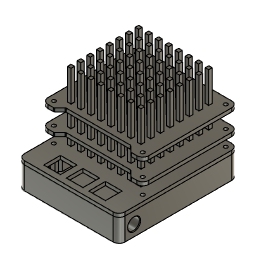
RGB-Audio-Visualiser (Autodesk Fusion 360 design; units mm, degrees)
Autodesk Fusion 360 part; units mm, degrees
sketch "Sketch1" plane through (0, 0, 0) normal (0, 0, 1) x (1, 0, 0) in component "Base"
  line L0 (-42.45, 0) -> (42.45, 0)
  line L1 (42.45, 0) -> (42.45, 100)
  line L2 (42.45, 100) -> (-42.45, 100)
  line L3 (-42.45, 100) -> (-42.45, 0)
  dimension "d18" = 84.9
  dimension "d19" = 100
  constraint horizontal L0
  constraint vertical L1
  constraint horizontal L2
  constraint vertical L3
  constraint midpoint origin L0
  measures "d18" distance of L0.start L0.end
  measures "d19" distance of L0.start L2.end
extrude "Extrude1" add sketch "Sketch1" along normal blind 19 makes body 1 in component "Base"
sketch "Sketch2" plane through (0, 0, 19) normal (0, 0, 1) x (-1, 0, 0) in component "Base"
  line L0 (42.45, -100) -> (42.45, 0)
  line L1 (42.45, 0) -> (-42.45, 0)
  line L2 (-42.45, 0) -> (-42.45, -100)
  line L3 (-42.45, -100) -> (42.45, -100)
  line L4 (33.45, -95) -> (-33.45, -95)
  line L5 (-33.45, -95) -> (-33.45, -5)
  line L6 (-33.45, -5) -> (33.45, -5)
  line L7 (33.45, -5) -> (33.45, -95)
  line L8 (0, -100) -> (0, 0) construction
  line L9 (30.95, -95) -> (-30.95, -95)
  line L10 (-30.95, -95) -> (-30.95, -45)
  line L11 (-33.45, -45) -> (33.45, -45)
  line L12 (30.95, -45) -> (30.95, -95)
  line L13 (-33.45, -21.9) -> (-35.05, -23.5)
  line L14 (-33.45, -21.9) -> (-30.5914, -21.9) construction
  line L15 (-35.05, -23.5) -> (-35.05, -26.5)
  line L16 (-35.05, -26.5) -> (-33.45, -28.1)
  line L17 (-35.05, -25) -> (-42.45, -25) construction
  line L18 (33.45, -21.9) -> (35.05, -23.5)
  line L19 (35.05, -23.5) -> (35.05, -26.5)
  line L20 (35.05, -26.5) -> (33.45, -28.1)
  line L21 (35.05, -25) -> (42.45, -25) construction
  line L22 (33.45, -92.95) -> (30.95, -92.95)
  line L23 (-30.95, -92.95) -> (-33.45, -92.95)
  dimension "d22" = 66.9
  dimension "d23" = 5
  dimension "d24" = 5
  dimension "d25" = 2.5
  dimension "d26" = 50
  dimension "d35" = 135
  dimension "d36" = 3
  dimension "d37" = 1.6
  dimension "d38" = 25
  dimension "d39" = 135
  dimension "d112" = 2.05
  constraint horizontal L4
  constraint vertical L5
  constraint horizontal L6
  constraint vertical L7
  constraint midpoint L3 L8.start
  constraint coincident L8.end origin
  constraint horizontal L9
  constraint vertical L10
  constraint horizontal L11
  constraint vertical L12
  constraint symmetric L8 L10 L12
  constraint collinear L4 L9
  constraint coincident L7 L11.end
  constraint coincident L12.start L11
  constraint coincident L5 L11.start
  constraint coincident L10.end L11
  constraint horizontal L14
  constraint coincident L5 L13.start
  constraint vertical L15
  constraint coincident L5 L16.end
  constraint equal L13 L16
  constraint midpoint L15 L17.start
  constraint coincident L2 L17.end
  constraint perpendicular L2 L17
  constraint coincident L7 L18.start
  constraint parallel L7 L19
  constraint coincident L7 L20.end
  constraint equal L18 L20
  constraint equal L13 L18
  constraint equal L15 L19
  constraint midpoint L19 L21.start
  constraint coincident L0 L21.end
  constraint perpendicular L0 L21
  constraint collinear L17 L21
  constraint coincident L7 L22.start
  constraint coincident L12 L22.end
  constraint perpendicular L12 L22
  constraint coincident L10 L23.start
  constraint coincident L5 L23.end
  constraint perpendicular L5 L23
  constraint collinear L22 L23
  measures "d22" distance of L4.start L4.end
  measures "d23" distance of L3 L4
  measures "d24" distance of L1 L6
  measures "d25" distance of L7 L12
  measures "d26" distance of L4 L11
  measures "d35" angle of L13 L14
  measures "d36" distance of L13.end L15.end
  measures "d37" distance of L5 L15
  measures "d38" distance of L1 L17
  measures "d39" angle of L18 L19
  measures "d112" distance of L4 L22.end
extrude "Extrude2" cut sketch "Sketch2" against normal blind 3.3 contours L4 L9 L10 L11 L12 | L7 L11 L12 L22 | L5 L6 L7 L11 | L5 L10 L11 L23 bodies 1 in component "Base"
extrude "Extrude3" cut sketch "Sketch2" against normal up to surface (17 mm away) contours L4 L9 L10 L11 L12 | L5 L6 L7 L11 | L7 L18 L19 L20 | L5 L13 L15 L16 bodies 1 in component "Base"
sketch "Sketch3" plane through (42.45, 0, 0) normal (1, 0, 0) x (0, 1, 0) in component "Base"
  line L0 (0, 0) -> (100, 0)
  line L1 (100, 0) -> (100, 19)
  line L2 (100, 19) -> (0, 19)
  line L3 (0, 19) -> (0, 0)
  circle A0 centre (12.7, 9.2) radius 5
  line L4 (5, 19) -> (5, 2)
  line L5 (5, 2) -> (21.9, 2)
  line L6 (28.1, 2) -> (45, 2)
  dimension "d31" = 10
  dimension "d32" = 7.7
  dimension "d65" = 7.2
  measures "d31" diameter of A0
  measures "d32" distance of A0.centre L4
  measures "d65" distance of A0.centre L5
extrude "Extrude4" cut sketch "Sketch3" against normal through all contours A0 bodies 1 in component "Base"
sketch "Sketch4" plane through (0, 100, 0) normal (0, 1, 0) x (-1, 0, 0) in component "Base"
  line L0 (-42.45, 0) -> (42.45, 0)
  line L1 (42.45, 0) -> (42.45, 19)
  line L2 (42.45, 19) -> (-42.45, 19)
  line L3 (-42.45, 19) -> (-42.45, 0)
  line L4 (-3.9, 6.1) -> (3.9, 6.1)
  line L5 (3.9, 6.1) -> (3.9, 2)
  line L6 (3.9, 2) -> (-3.9, 2)
  line L7 (-3.9, 2) -> (-3.9, 6.1)
  line L8 (0, 19) -> (0, 0) construction
  line L9 (-30.95, 2) -> (30.95, 2)
  line L10 (-5.9, 0) -> (-5.9, 8.3)
  line L11 (-5.9, 8.3) -> (5.9, 8.3)
  line L12 (5.9, 8.3) -> (5.9, 0)
  dimension "d40" = 7.8
  dimension "d41" = 4.1
  dimension "d115" = 2
  dimension "d116" = 2.2
  constraint horizontal L4
  constraint vertical L5
  constraint horizontal L6
  constraint vertical L7
  constraint midpoint L2 L8.start
  constraint coincident L8.end origin
  constraint symmetric L5 L7 L8
  constraint collinear L6 L9
  constraint coincident L0 L10.start
  constraint perpendicular L0 L10
  constraint perpendicular L10 L11
  constraint coincident L0 L12.end
  constraint perpendicular L0 L12
  constraint symmetric L8 L10 L12
  measures "d40" distance of L4.start L4.end
  measures "d41" distance of L4.start L6.end
  measures "d115" distance of L7 L10
  measures "d116" distance of L4 L11
extrude "Extrude5" cut sketch "Sketch4" against normal blind 2 contours L0 L6 L9 L10 L12 | L4 L5 L7 L9 L10 L11 L12 | L4 L5 L6 L7 L9 bodies 1 in component "Base"
extrude "Extrude6" cut sketch "Sketch4" against normal up to surface (5 mm away) contours L4 L5 L6 L7 L9 bodies 1 in component "Base"
sketch "Sketch5" plane through (0, 0, 0) normal (1, 0, 0) x (0, 1, 0) in component "Base"
  line L0 (48, 2) -> (52, 2)
  line L1 (52, 2) -> (52, 9.4)
  line L2 (52, 9.4) -> (48, 9.4)
  line L3 (48, 9.4) -> (48, 2)
  line L4 (95, 2) -> (45, 2)
  line L5 (52, 7.9) -> (52, 9.4)
  line L6 (52, 6) -> (56.5, 6)
  line L7 (56.5, 6) -> (56.5, 2)
  line L8 (56.5, 2) -> (52, 2)
  line L9 (52, 2) -> (52, 6)
  line L10 (95, 19) -> (95, 2)
  dimension "d49" = 4
  dimension "d50" = 4.5
  dimension "d51" = 43
  dimension "d113" = 4
  dimension "d114" = 7.4
  constraint horizontal L0
  constraint vertical L1
  constraint horizontal L2
  constraint vertical L3
  constraint coincident L0.start L4
  constraint vertical L5
  constraint horizontal L6
  constraint vertical L7
  constraint horizontal L8
  constraint vertical L9
  constraint coincident L4 L7.end
  constraint coincident L1 L6.start
  measures "d49" distance of L6.end L7.end
  measures "d50" distance of L1 L7
  measures "d51" distance of L1 L10
  measures "d113" distance of L1.end L2.end
  measures "d114" distance of L0.start L2.end
extrude "Extrude7" add sketch "Sketch5" along normal mid plane 9 bodies 1 in component "Base"
fillet "Fillet1" radius 5 4 edges at (42.45, 0, 9.5) (42.45, 100, 9.5) (-42.45, 0, 9.5) (-42.45, 100, 9.5) on bodies 1 in component "Base"
fillet "Fillet1" radius 0.5 22 edges at (-33.45, 5, 10.5) (33.45, 5, 10.5) (4.5, 48, 5.7) (4.5, 56.5, 4) (-4.5, 48, 5.7) (-4.5, 56.5, 4) (-4.5, 52, 7.7) (4.5, 52, 7.7) (42.45, 8.0384, 11.0081) (-33.45, 8.0384, 11.0081) (-42.45, 8.0384, 7.3919) (33.45, 8.0384, 7.3919) (-3.9, 95, 4.05) (-3.9, 98, 4.05) (3.9, 95, 4.05) (3.9, 98, 4.05) (-33.45, 92.95, 17.35) (33.45, 92.95, 17.35) (5.9, 100, 4.15) (-5.9, 100, 4.15) (5.9, 98, 4.15) (-5.9, 98, 4.15) on bodies 1 in component "Base"
chamfer "Chamfer1" distance 2.5 angle 45 4 edges at (-30.95, 45, 8.85) (-30.95, 95, 10.5) (30.95, 95, 10.5) (30.95, 45, 8.85) on bodies 1 in component "Base"
sketch "Sketch7" plane through (0, 0, 0) normal (0, 0, -1) x (1, 0, 0) in component "Base"
  arc A0 (-42.45, -95) -> (-37.45, -100) centre (-37.45, -95) ccw
  line L0 (-37.45, -100) -> (-6.4, -100)
  line L1 (-5.4, -98) -> (5.4, -98)
  line L2 (6.4, -100) -> (37.45, -100)
  arc A1 (37.45, -100) -> (42.45, -95) centre (37.45, -95) ccw
  line L3 (42.45, -95) -> (42.45, -5)
  arc A2 (42.45, -5) -> (37.45, 0) centre (37.45, -5) ccw
  line L4 (37.45, 0) -> (-37.45, 0)
  arc A3 (-37.45, 0) -> (-42.45, -5) centre (-37.45, -5) ccw
  line L5 (-42.45, -5) -> (-42.45, -95)
  line L6 (-5.9, -99.5) -> (-5.9, -98.5)
  line L7 (5.9, -98.5) -> (5.9, -99.5)
  arc A4 (-6.4, -100) -> (-5.9, -99.5) centre (-6.4, -99.5) ccw
  arc A5 (-5.4, -98) -> (-5.9, -98.5) centre (-5.4, -98.5) ccw
  arc A6 (5.9, -98.5) -> (5.4, -98) centre (5.4, -98.5) ccw
  arc A7 (5.9, -99.5) -> (6.4, -100) centre (6.4, -99.5) ccw
  point P0 (-37.45, -95)
  point P1 (37.45, -95)
  point P2 (-37.45, -25)
  point P3 (37.45, -25)
  dimension "d66" = 25
  constraint coincident P0 A0.centre
  constraint coincident P1 A1.centre
  constraint horizontal P2 P3
  constraint vertical P0 P2
  constraint vertical P1 P3
  measures "d66" distance of L4 P2
hole "Hole2" at (37.45, 25, 0) at (37.45, 95, 0) at (-37.45, 95, 0) at (-37.45, 25, 0) direction (0, 0, 1) diameter 3.1 end through all counterbore diameter 6 counterbore depth 2 bodies 1 in component "Base"
sketch "Sketch1 (2)" plane through (0, 0, 19) normal (0, 0, 1) x (-1, 0, 0) in component "Cover"
  circle A0 centre (37.45, -95) radius 1.55
  circle A1 centre (-37.45, -25) radius 1.55
  circle A2 centre (-37.45, -95) radius 1.55
  circle A3 centre (37.45, -25) radius 1.55
  arc A4 (37.45, -100) -> (42.45, -95) centre (37.45, -95) ccw
  line L0 (42.45, -95) -> (42.45, -5)
  arc A5 (42.45, -5) -> (37.45, 0) centre (37.45, -5) ccw
  line L1 (37.45, 0) -> (-37.45, 0)
  arc A6 (-37.45, 0) -> (-42.45, -5) centre (-37.45, -5) ccw
  line L2 (-42.45, -5) -> (-42.45, -95)
  arc A7 (-42.45, -95) -> (-37.45, -100) centre (-37.45, -95) ccw
  line L3 (-37.45, -100) -> (37.45, -100)
  line L4 (33.45, -21.9) -> (35.05, -23.5)
  line L5 (35.05, -23.5) -> (35.05, -26.5)
  line L6 (35.05, -26.5) -> (33.45, -28.1)
  line L7 (33.45, -28.1) -> (33.45, -92.45)
  line L8 (28.45, -95) -> (-28.45, -95)
  line L9 (-33.45, -92.45) -> (-33.45, -28.1)
  line L10 (-33.45, -28.1) -> (-35.05, -26.5)
  line L11 (-35.05, -26.5) -> (-35.05, -23.5)
  line L12 (-35.05, -23.5) -> (-33.45, -21.9)
  line L13 (-33.45, -21.9) -> (-33.45, -5.5)
  arc A8 (-32.95, -5) -> (-33.45, -5.5) centre (-32.95, -5.5) ccw
  line L14 (-32.95, -5) -> (32.95, -5)
  arc A9 (33.45, -5.5) -> (32.95, -5) centre (32.95, -5.5) ccw
  line L15 (33.45, -5.5) -> (33.45, -21.9)
  line L16 (32.95, -92.95) -> (30.5, -92.95)
  line L17 (30.5, -92.95) -> (28.45, -95)
  line L18 (-28.45, -95) -> (-30.5, -92.95)
  line L19 (-30.5, -92.95) -> (-32.95, -92.95)
  arc A10 (32.95, -92.95) -> (33.45, -92.45) centre (32.95, -92.45) ccw
  arc A11 (-33.45, -92.45) -> (-32.95, -92.95) centre (-32.95, -92.45) ccw
extrude "Extrude1'" add sketch "Sketch1 (2)" along normal blind 3 separate body contours A4 L0 A5 L1 A6 L2 A7 L3 | L4 L5 L6 L7 L8 L9 L10 L11 L12 L13 A8 L14 A9 L15 L16 L17 L18 L19 A10 A11 makes body 2 in component "Cover"
sketch "Sketch2 (2)" plane through (0, 0, 22) normal (0, 0, 1) x (-1, 0, 0) in component "Cover"
  circle A0 centre (-37.45, -25) radius 1.55
  circle A1 centre (-37.45, -95) radius 1.55
  circle A2 centre (37.45, -25) radius 1.55
  circle A3 centre (37.45, -95) radius 1.55
  line L0 (-37.45, -100) -> (37.45, -100)
  arc A4 (37.45, -100) -> (42.45, -95) centre (37.45, -95) ccw
  line L1 (42.45, -95) -> (42.45, -5)
  arc A5 (42.45, -5) -> (37.45, 0) centre (37.45, -5) ccw
  line L2 (37.45, 0) -> (-37.45, 0)
  arc A6 (-37.45, 0) -> (-42.45, -5) centre (-37.45, -5) ccw
  line L3 (-42.45, -5) -> (-42.45, -95)
  arc A7 (-42.45, -95) -> (-37.45, -100) centre (-37.45, -95) ccw
  line L4 (0, -100) -> (0, 0) construction
  line L5 (7, -5) -> (-7, -5)
  line L6 (-7, -5) -> (-7, -19)
  line L7 (-7, -19) -> (7, -19)
  line L8 (7, -19) -> (7, -5)
  line L9 (31.85, -90.85) -> (-31.85, -90.85) construction
  line L10 (-31.85, -90.85) -> (-31.85, -29.15) construction
  line L11 (-31.85, -29.15) -> (31.85, -29.15) construction
  line L12 (31.85, -29.15) -> (31.85, -90.85) construction
  line L13 (37.45, -95) -> (-37.45, -25) construction
  line L14 (-31.85, -90.85) -> (31.85, -29.15) construction
  line L15 (31, -90) -> (28, -90)
  line L16 (28, -90) -> (28, -87)
  line L17 (28, -87) -> (31, -87)
  line L18 (31, -87) -> (31, -90)
  dimension "d77" = 14
  dimension "d78" = 5
  dimension "d79" = 63.7
  dimension "d80" = 61.7
  dimension "d81" = 3
  dimension "d82" = 0.85
  dimension "d83" = 0.85
  constraint midpoint L0 L4.start
  constraint coincident L4.end origin
  constraint horizontal L5
  constraint vertical L6
  constraint horizontal L7
  constraint vertical L8
  constraint equal L5 L8
  constraint symmetric L4 L6 L8
  constraint horizontal L9
  constraint vertical L10
  constraint horizontal L11
  constraint vertical L12
  constraint coincident A3.centre A4.centre
  constraint coincident A0.centre L13.end
  constraint midpoint L13 L14
  constraint horizontal L15
  constraint vertical L16
  constraint horizontal L17
  constraint vertical L18
  constraint equal L15 L18
  measures "d77" distance of L5.start L5.end
  measures "d78" distance of L2 L5
  measures "d79" distance of L9.start L9.end
  measures "d80" distance of L9.end L10.end
  measures "d81" distance of L15.start L15.end
  measures "d82" distance of L9 L15
  measures "d83" distance of L12 L18
extrude "Extrude2'" cut sketch "Sketch2 (2)" against normal through all contours L5 L6 L7 L8 bodies 2 in component "Cover"
pattern_linear "R-Pattern1" count 3 spacing 19 along (-1, 0, 0) both ways of "Extrude2'" in component "Cover"
extrude "Extrude3'" cut sketch "Sketch2 (2)" against normal through all contours L15 L16 L17 L18 bodies 2 in component "Cover"
pattern_linear "R-Pattern2" count 8 spacing 8.4286 along (1, 0, 0) count 8 spacing 8.1429 along (0, -1, 0) of "Extrude3'" in component "Cover"
ref_plane "WorkPlane1" through (0, 50, 32) normal (0, 0, 1) x (-1, 0, 0) in component "Layer"
sketch "Sketch1 (3)" plane through (0, 50, 32) normal (0, 0, 1) x (1, 0, 0) in component "Layer"
  line L0 (28, -20) -> (28, -17)
  line L1 (28, -17) -> (31, -17)
  line L2 (31, -17) -> (31, -20)
  line L3 (31, -20) -> (28, -20)
  line L4 (19.5714, -20) -> (19.5714, -17)
  line L5 (19.5714, -17) -> (22.5714, -17)
  line L6 (22.5714, -17) -> (22.5714, -20)
  line L7 (22.5714, -20) -> (19.5714, -20)
  line L8 (11.1429, -20) -> (11.1429, -17)
  line L9 (11.1429, -17) -> (14.1429, -17)
  line L10 (14.1429, -17) -> (14.1429, -20)
  line L11 (14.1429, -20) -> (11.1429, -20)
  line L12 (2.7143, -20) -> (2.7143, -17)
  line L13 (2.7143, -17) -> (5.7143, -17)
  line L14 (5.7143, -17) -> (5.7143, -20)
  line L15 (5.7143, -20) -> (2.7143, -20)
  line L16 (-5.7143, -20) -> (-5.7143, -17)
  line L17 (-5.7143, -17) -> (-2.7143, -17)
  line L18 (-2.7143, -17) -> (-2.7143, -20)
  line L19 (-2.7143, -20) -> (-5.7143, -20)
  line L20 (-14.1429, -20) -> (-14.1429, -17)
  line L21 (-14.1429, -17) -> (-11.1429, -17)
  line L22 (-11.1429, -17) -> (-11.1429, -20)
  line L23 (-11.1429, -20) -> (-14.1429, -20)
  line L24 (-22.5714, -20) -> (-22.5714, -17)
  line L25 (-22.5714, -17) -> (-19.5714, -17)
  line L26 (-19.5714, -17) -> (-19.5714, -20)
  line L27 (-19.5714, -20) -> (-22.5714, -20)
  line L28 (-31, -20) -> (-31, -17)
  line L29 (-31, -17) -> (-28, -17)
  line L30 (-28, -17) -> (-28, -20)
  line L31 (-28, -20) -> (-31, -20)
  line L32 (28, -11.8571) -> (28, -8.8571)
  line L33 (28, -8.8571) -> (31, -8.8571)
  line L34 (31, -8.8571) -> (31, -11.8571)
  line L35 (31, -11.8571) -> (28, -11.8571)
  line L36 (19.5714, -11.8571) -> (19.5714, -8.8571)
  line L37 (19.5714, -8.8571) -> (22.5714, -8.8571)
  line L38 (22.5714, -8.8571) -> (22.5714, -11.8571)
  line L39 (22.5714, -11.8571) -> (19.5714, -11.8571)
  line L40 (11.1429, -11.8571) -> (11.1429, -8.8571)
  line L41 (11.1429, -8.8571) -> (14.1429, -8.8571)
  line L42 (14.1429, -8.8571) -> (14.1429, -11.8571)
  line L43 (14.1429, -11.8571) -> (11.1429, -11.8571)
  line L44 (2.7143, -11.8571) -> (2.7143, -8.8571)
  line L45 (2.7143, -8.8571) -> (5.7143, -8.8571)
  line L46 (5.7143, -8.8571) -> (5.7143, -11.8571)
  line L47 (5.7143, -11.8571) -> (2.7143, -11.8571)
  line L48 (-5.7143, -11.8571) -> (-5.7143, -8.8571)
  line L49 (-5.7143, -8.8571) -> (-2.7143, -8.8571)
  line L50 (-2.7143, -8.8571) -> (-2.7143, -11.8571)
  line L51 (-2.7143, -11.8571) -> (-5.7143, -11.8571)
  line L52 (-14.1429, -11.8571) -> (-14.1429, -8.8571)
  line L53 (-14.1429, -8.8571) -> (-11.1429, -8.8571)
  line L54 (-11.1429, -8.8571) -> (-11.1429, -11.8571)
  line L55 (-11.1429, -11.8571) -> (-14.1429, -11.8571)
  line L56 (-22.5714, -11.8571) -> (-22.5714, -8.8571)
  line L57 (-22.5714, -8.8571) -> (-19.5714, -8.8571)
  line L58 (-19.5714, -8.8571) -> (-19.5714, -11.8571)
  line L59 (-19.5714, -11.8571) -> (-22.5714, -11.8571)
  line L60 (-31, -11.8571) -> (-31, -8.8571)
  line L61 (-31, -8.8571) -> (-28, -8.8571)
  line L62 (-28, -8.8571) -> (-28, -11.8571)
  line L63 (-28, -11.8571) -> (-31, -11.8571)
  line L64 (28, -3.7143) -> (28, -0.7143)
  line L65 (28, -0.7143) -> (31, -0.7143)
  line L66 (31, -0.7143) -> (31, -3.7143)
  line L67 (31, -3.7143) -> (28, -3.7143)
  line L68 (19.5714, -3.7143) -> (19.5714, -0.7143)
  line L69 (19.5714, -0.7143) -> (22.5714, -0.7143)
  line L70 (22.5714, -0.7143) -> (22.5714, -3.7143)
  line L71 (22.5714, -3.7143) -> (19.5714, -3.7143)
  line L72 (11.1429, -3.7143) -> (11.1429, -0.7143)
  line L73 (11.1429, -0.7143) -> (14.1429, -0.7143)
  line L74 (14.1429, -0.7143) -> (14.1429, -3.7143)
  line L75 (14.1429, -3.7143) -> (11.1429, -3.7143)
  line L76 (2.7143, -3.7143) -> (2.7143, -0.7143)
  line L77 (2.7143, -0.7143) -> (5.7143, -0.7143)
  line L78 (5.7143, -0.7143) -> (5.7143, -3.7143)
  line L79 (5.7143, -3.7143) -> (2.7143, -3.7143)
  line L80 (-5.7143, -3.7143) -> (-5.7143, -0.7143)
  line L81 (-5.7143, -0.7143) -> (-2.7143, -0.7143)
  line L82 (-2.7143, -0.7143) -> (-2.7143, -3.7143)
  line L83 (-2.7143, -3.7143) -> (-5.7143, -3.7143)
  line L84 (-14.1429, -3.7143) -> (-14.1429, -0.7143)
  line L85 (-14.1429, -0.7143) -> (-11.1429, -0.7143)
  line L86 (-11.1429, -0.7143) -> (-11.1429, -3.7143)
  line L87 (-11.1429, -3.7143) -> (-14.1429, -3.7143)
  line L88 (-22.5714, -3.7143) -> (-22.5714, -0.7143)
  line L89 (-22.5714, -0.7143) -> (-19.5714, -0.7143)
  line L90 (-19.5714, -0.7143) -> (-19.5714, -3.7143)
  line L91 (-19.5714, -3.7143) -> (-22.5714, -3.7143)
  line L92 (-31, -3.7143) -> (-31, -0.7143)
  line L93 (-31, -0.7143) -> (-28, -0.7143)
  line L94 (-28, -0.7143) -> (-28, -3.7143)
  line L95 (-28, -3.7143) -> (-31, -3.7143)
  line L96 (28, 4.4286) -> (28, 7.4286)
  line L97 (28, 7.4286) -> (31, 7.4286)
  line L98 (31, 7.4286) -> (31, 4.4286)
  line L99 (31, 4.4286) -> (28, 4.4286)
  line L100 (19.5714, 4.4286) -> (19.5714, 7.4286)
  line L101 (19.5714, 7.4286) -> (22.5714, 7.4286)
  line L102 (22.5714, 7.4286) -> (22.5714, 4.4286)
  line L103 (22.5714, 4.4286) -> (19.5714, 4.4286)
  line L104 (11.1429, 4.4286) -> (11.1429, 7.4286)
  line L105 (11.1429, 7.4286) -> (14.1429, 7.4286)
  line L106 (14.1429, 7.4286) -> (14.1429, 4.4286)
  line L107 (14.1429, 4.4286) -> (11.1429, 4.4286)
  line L108 (2.7143, 4.4286) -> (2.7143, 7.4286)
  line L109 (2.7143, 7.4286) -> (5.7143, 7.4286)
  line L110 (5.7143, 7.4286) -> (5.7143, 4.4286)
  line L111 (5.7143, 4.4286) -> (2.7143, 4.4286)
  line L112 (-5.7143, 4.4286) -> (-5.7143, 7.4286)
  line L113 (-5.7143, 7.4286) -> (-2.7143, 7.4286)
  line L114 (-2.7143, 7.4286) -> (-2.7143, 4.4286)
  line L115 (-2.7143, 4.4286) -> (-5.7143, 4.4286)
  line L116 (-14.1429, 4.4286) -> (-14.1429, 7.4286)
  line L117 (-14.1429, 7.4286) -> (-11.1429, 7.4286)
  line L118 (-11.1429, 7.4286) -> (-11.1429, 4.4286)
  line L119 (-11.1429, 4.4286) -> (-14.1429, 4.4286)
  line L120 (-22.5714, 4.4286) -> (-22.5714, 7.4286)
  line L121 (-22.5714, 7.4286) -> (-19.5714, 7.4286)
  line L122 (-19.5714, 7.4286) -> (-19.5714, 4.4286)
  line L123 (-19.5714, 4.4286) -> (-22.5714, 4.4286)
  line L124 (-31, 4.4286) -> (-31, 7.4286)
  line L125 (-31, 7.4286) -> (-28, 7.4286)
  line L126 (-28, 7.4286) -> (-28, 4.4286)
  line L127 (-28, 4.4286) -> (-31, 4.4286)
  line L128 (28, 12.5714) -> (28, 15.5714)
  line L129 (28, 15.5714) -> (31, 15.5714)
  line L130 (31, 15.5714) -> (31, 12.5714)
  line L131 (31, 12.5714) -> (28, 12.5714)
  line L132 (19.5714, 12.5714) -> (19.5714, 15.5714)
  line L133 (19.5714, 15.5714) -> (22.5714, 15.5714)
  line L134 (22.5714, 15.5714) -> (22.5714, 12.5714)
  line L135 (22.5714, 12.5714) -> (19.5714, 12.5714)
  line L136 (11.1429, 12.5714) -> (11.1429, 15.5714)
  line L137 (11.1429, 15.5714) -> (14.1429, 15.5714)
  line L138 (14.1429, 15.5714) -> (14.1429, 12.5714)
  line L139 (14.1429, 12.5714) -> (11.1429, 12.5714)
  line L140 (2.7143, 12.5714) -> (2.7143, 15.5714)
  line L141 (2.7143, 15.5714) -> (5.7143, 15.5714)
  line L142 (5.7143, 15.5714) -> (5.7143, 12.5714)
  line L143 (5.7143, 12.5714) -> (2.7143, 12.5714)
  line L144 (-5.7143, 12.5714) -> (-5.7143, 15.5714)
  line L145 (-5.7143, 15.5714) -> (-2.7143, 15.5714)
  line L146 (-2.7143, 15.5714) -> (-2.7143, 12.5714)
  line L147 (-2.7143, 12.5714) -> (-5.7143, 12.5714)
  line L148 (-14.1429, 12.5714) -> (-14.1429, 15.5714)
  line L149 (-14.1429, 15.5714) -> (-11.1429, 15.5714)
  line L150 (-11.1429, 15.5714) -> (-11.1429, 12.5714)
  line L151 (-11.1429, 12.5714) -> (-14.1429, 12.5714)
  line L152 (-22.5714, 12.5714) -> (-22.5714, 15.5714)
  line L153 (-22.5714, 15.5714) -> (-19.5714, 15.5714)
  line L154 (-19.5714, 15.5714) -> (-19.5714, 12.5714)
  line L155 (-19.5714, 12.5714) -> (-22.5714, 12.5714)
  line L156 (-31, 12.5714) -> (-31, 15.5714)
  line L157 (-31, 15.5714) -> (-28, 15.5714)
  line L158 (-28, 15.5714) -> (-28, 12.5714)
  line L159 (-28, 12.5714) -> (-31, 12.5714)
  line L160 (28, 20.7143) -> (28, 23.7143)
  line L161 (28, 23.7143) -> (31, 23.7143)
  line L162 (31, 23.7143) -> (31, 20.7143)
  line L163 (31, 20.7143) -> (28, 20.7143)
  line L164 (19.5714, 20.7143) -> (19.5714, 23.7143)
  line L165 (19.5714, 23.7143) -> (22.5714, 23.7143)
  line L166 (22.5714, 23.7143) -> (22.5714, 20.7143)
  line L167 (22.5714, 20.7143) -> (19.5714, 20.7143)
  line L168 (11.1429, 20.7143) -> (11.1429, 23.7143)
  line L169 (11.1429, 23.7143) -> (14.1429, 23.7143)
  line L170 (14.1429, 23.7143) -> (14.1429, 20.7143)
  line L171 (14.1429, 20.7143) -> (11.1429, 20.7143)
  line L172 (2.7143, 20.7143) -> (2.7143, 23.7143)
  line L173 (2.7143, 23.7143) -> (5.7143, 23.7143)
  line L174 (5.7143, 23.7143) -> (5.7143, 20.7143)
  line L175 (5.7143, 20.7143) -> (2.7143, 20.7143)
  line L176 (-5.7143, 20.7143) -> (-5.7143, 23.7143)
  line L177 (-5.7143, 23.7143) -> (-2.7143, 23.7143)
  line L178 (-2.7143, 23.7143) -> (-2.7143, 20.7143)
  line L179 (-2.7143, 20.7143) -> (-5.7143, 20.7143)
  line L180 (-14.1429, 20.7143) -> (-14.1429, 23.7143)
  line L181 (-14.1429, 23.7143) -> (-11.1429, 23.7143)
  line L182 (-11.1429, 23.7143) -> (-11.1429, 20.7143)
  line L183 (-11.1429, 20.7143) -> (-14.1429, 20.7143)
  line L184 (-22.5714, 20.7143) -> (-22.5714, 23.7143)
  line L185 (-22.5714, 23.7143) -> (-19.5714, 23.7143)
  line L186 (-19.5714, 23.7143) -> (-19.5714, 20.7143)
  line L187 (-19.5714, 20.7143) -> (-22.5714, 20.7143)
  line L188 (-31, 20.7143) -> (-31, 23.7143)
  line L189 (-31, 23.7143) -> (-28, 23.7143)
  line L190 (-28, 23.7143) -> (-28, 20.7143)
  line L191 (-28, 20.7143) -> (-31, 20.7143)
  line L192 (28, 28.8571) -> (28, 31.8571)
  line L193 (28, 31.8571) -> (31, 31.8571)
  line L194 (31, 31.8571) -> (31, 28.8571)
  line L195 (31, 28.8571) -> (28, 28.8571)
  line L196 (19.5714, 28.8571) -> (19.5714, 31.8571)
  line L197 (19.5714, 31.8571) -> (22.5714, 31.8571)
  line L198 (22.5714, 31.8571) -> (22.5714, 28.8571)
  line L199 (22.5714, 28.8571) -> (19.5714, 28.8571)
  line L200 (11.1429, 28.8571) -> (11.1429, 31.8571)
  line L201 (11.1429, 31.8571) -> (14.1429, 31.8571)
  line L202 (14.1429, 31.8571) -> (14.1429, 28.8571)
  line L203 (14.1429, 28.8571) -> (11.1429, 28.8571)
  line L204 (2.7143, 28.8571) -> (2.7143, 31.8571)
  line L205 (2.7143, 31.8571) -> (5.7143, 31.8571)
  line L206 (5.7143, 31.8571) -> (5.7143, 28.8571)
  line L207 (5.7143, 28.8571) -> (2.7143, 28.8571)
  line L208 (-5.7143, 28.8571) -> (-5.7143, 31.8571)
  line L209 (-5.7143, 31.8571) -> (-2.7143, 31.8571)
  line L210 (-2.7143, 31.8571) -> (-2.7143, 28.8571)
  line L211 (-2.7143, 28.8571) -> (-5.7143, 28.8571)
  line L212 (-14.1429, 28.8571) -> (-14.1429, 31.8571)
  line L213 (-14.1429, 31.8571) -> (-11.1429, 31.8571)
  line L214 (-11.1429, 31.8571) -> (-11.1429, 28.8571)
  line L215 (-11.1429, 28.8571) -> (-14.1429, 28.8571)
  line L216 (-22.5714, 28.8571) -> (-22.5714, 31.8571)
  line L217 (-22.5714, 31.8571) -> (-19.5714, 31.8571)
  line L218 (-19.5714, 31.8571) -> (-19.5714, 28.8571)
  line L219 (-19.5714, 28.8571) -> (-22.5714, 28.8571)
  line L220 (-31, 28.8571) -> (-31, 31.8571)
  line L221 (-31, 31.8571) -> (-28, 31.8571)
  line L222 (-28, 31.8571) -> (-28, 28.8571)
  line L223 (-28, 28.8571) -> (-31, 28.8571)
  line L224 (28, 37) -> (28, 40)
  line L225 (28, 40) -> (31, 40)
  line L226 (31, 40) -> (31, 37)
  line L227 (31, 37) -> (28, 37)
  line L228 (19.5714, 37) -> (19.5714, 40)
  line L229 (19.5714, 40) -> (22.5714, 40)
  line L230 (22.5714, 40) -> (22.5714, 37)
  line L231 (22.5714, 37) -> (19.5714, 37)
  line L232 (11.1429, 37) -> (11.1429, 40)
  line L233 (11.1429, 40) -> (14.1429, 40)
  line L234 (14.1429, 40) -> (14.1429, 37)
  line L235 (14.1429, 37) -> (11.1429, 37)
  line L236 (2.7143, 37) -> (2.7143, 40)
  line L237 (2.7143, 40) -> (5.7143, 40)
  line L238 (5.7143, 40) -> (5.7143, 37)
  line L239 (5.7143, 37) -> (2.7143, 37)
  line L240 (-5.7143, 37) -> (-5.7143, 40)
  line L241 (-5.7143, 40) -> (-2.7143, 40)
  line L242 (-2.7143, 40) -> (-2.7143, 37)
  line L243 (-2.7143, 37) -> (-5.7143, 37)
  line L244 (-14.1429, 37) -> (-14.1429, 40)
  line L245 (-14.1429, 40) -> (-11.1429, 40)
  line L246 (-11.1429, 40) -> (-11.1429, 37)
  line L247 (-11.1429, 37) -> (-14.1429, 37)
  line L248 (-22.5714, 37) -> (-22.5714, 40)
  line L249 (-22.5714, 40) -> (-19.5714, 40)
  line L250 (-19.5714, 40) -> (-19.5714, 37)
  line L251 (-19.5714, 37) -> (-22.5714, 37)
  line L252 (-31, 37) -> (-31, 40)
  line L253 (-31, 40) -> (-28, 40)
  line L254 (-28, 40) -> (-28, 37)
  line L255 (-28, 37) -> (-31, 37)
  line L256 (-26, -31) -> (-12, -31)
  line L257 (-12, -31) -> (-12, -45)
  line L258 (-12, -45) -> (-26, -45)
  line L259 (-26, -45) -> (-26, -31)
  line L260 (12, -31) -> (26, -31)
  line L261 (26, -31) -> (26, -45)
  line L262 (26, -45) -> (12, -45)
  line L263 (12, -45) -> (12, -31)
  line L264 (-7, -31) -> (7, -31)
  line L265 (7, -31) -> (7, -45)
  line L266 (7, -45) -> (-7, -45)
  line L267 (-7, -45) -> (-7, -31)
  circle A0 centre (37.45, -25) radius 1.55
  circle A1 centre (37.45, 45) radius 1.55
  circle A2 centre (-37.45, -25) radius 1.55
  circle A3 centre (-37.45, 45) radius 1.55
  line L268 (37.45, 50) -> (-37.45, 50)
  arc A4 (-37.45, 50) -> (-42.45, 45) centre (-37.45, 45) ccw
  line L269 (-42.45, 45) -> (-42.45, -45)
  arc A5 (-42.45, -45) -> (-37.45, -50) centre (-37.45, -45) ccw
  line L270 (-37.45, -50) -> (37.45, -50)
  arc A6 (37.45, -50) -> (42.45, -45) centre (37.45, -45) ccw
  line L271 (42.45, -45) -> (42.45, 45)
  arc A7 (42.45, 45) -> (37.45, 50) centre (37.45, 45) ccw
  line L272 (-42.45, -30) -> (-32.45, -30)
  line L273 (-32.45, -30) -> (-27.45, -25)
  line L274 (-27.45, -25) -> (27.45, -25)
  line L275 (27.45, -25) -> (32.45, -30)
  line L276 (32.45, -30) -> (42.45, -30)
  dimension "d98" = 5
  dimension "d99" = 135
  dimension "d100" = 5
  constraint coincident L269 L272.start
  constraint perpendicular L269 L272
  constraint perpendicular L269 L274
  constraint coincident L271 L276.end
  constraint perpendicular L271 L276
  constraint equal L272 L276
  constraint equal L273 L275
  constraint collinear L272 L276
  constraint horizontal A2.centre L273.end
  measures "d98" distance of A2.centre L272
  measures "d99" angle of L273 L274
  measures "d100" horizontal distance of A2.centre L272.end
extrude "Extrude1''" add sketch "Sketch1 (3)" along normal blind 3 separate body contours L268 A4 L269 L271 A7 L272 L273 L274 L275 L276 makes body 3 in component "Layer"
fillet "Fillet1'" radius 5 2 edges at (-42.45, 20, 33.5) (42.45, 20, 33.5) on bodies 3 in component "Layer"
fillet "Fillet1'" radius 1 4 edges at (32.45, 20, 33.5) (-32.45, 20, 33.5) (-27.45, 25, 33.5) (27.45, 25, 33.5) on bodies 3 in component "Layer"
extrude "Extrude1'''" add 1 faces at (-38.6333, 59.1429, 35) along direction (0, 0, 1) blind 3 from surface at 15 separate body on bodies 3 makes body 4 in component "Top"
sketch "Sketch1 (4)" plane through (0, 0, 19) normal (0, 0, -1) x (1, 0, 0) in component "Light Sticks"
  line L0 (28, -33) -> (28, -30)
  line L1 (28, -30) -> (31, -30)
  line L2 (31, -30) -> (31, -33)
  line L3 (31, -33) -> (28, -33)
  line L4 (19.5714, -33) -> (19.5714, -30)
  line L5 (19.5714, -30) -> (22.5714, -30)
  line L6 (22.5714, -30) -> (22.5714, -33)
  line L7 (22.5714, -33) -> (19.5714, -33)
  line L8 (11.1429, -33) -> (11.1429, -30)
  line L9 (11.1429, -30) -> (14.1429, -30)
  line L10 (14.1429, -30) -> (14.1429, -33)
  line L11 (14.1429, -33) -> (11.1429, -33)
  line L12 (2.7143, -33) -> (2.7143, -30)
  line L13 (2.7143, -30) -> (5.7143, -30)
  line L14 (5.7143, -30) -> (5.7143, -33)
  line L15 (5.7143, -33) -> (2.7143, -33)
  line L16 (-5.7143, -33) -> (-5.7143, -30)
  line L17 (-5.7143, -30) -> (-2.7143, -30)
  line L18 (-2.7143, -30) -> (-2.7143, -33)
  line L19 (-2.7143, -33) -> (-5.7143, -33)
  line L20 (-14.1429, -33) -> (-14.1429, -30)
  line L21 (-14.1429, -30) -> (-11.1429, -30)
  line L22 (-11.1429, -30) -> (-11.1429, -33)
  line L23 (-11.1429, -33) -> (-14.1429, -33)
  line L24 (-22.5714, -33) -> (-22.5714, -30)
  line L25 (-22.5714, -30) -> (-19.5714, -30)
  line L26 (-19.5714, -30) -> (-19.5714, -33)
  line L27 (-19.5714, -33) -> (-22.5714, -33)
  line L28 (-31, -33) -> (-31, -30)
  line L29 (-31, -30) -> (-28, -30)
  line L30 (-28, -30) -> (-28, -33)
  line L31 (-28, -33) -> (-31, -33)
  line L32 (28, -41.1429) -> (28, -38.1429)
  line L33 (28, -38.1429) -> (31, -38.1429)
  line L34 (31, -38.1429) -> (31, -41.1429)
  line L35 (31, -41.1429) -> (28, -41.1429)
  line L36 (19.5714, -41.1429) -> (19.5714, -38.1429)
  line L37 (19.5714, -38.1429) -> (22.5714, -38.1429)
  line L38 (22.5714, -38.1429) -> (22.5714, -41.1429)
  line L39 (22.5714, -41.1429) -> (19.5714, -41.1429)
  line L40 (11.1429, -41.1429) -> (11.1429, -38.1429)
  line L41 (11.1429, -38.1429) -> (14.1429, -38.1429)
  line L42 (14.1429, -38.1429) -> (14.1429, -41.1429)
  line L43 (14.1429, -41.1429) -> (11.1429, -41.1429)
  line L44 (2.7143, -41.1429) -> (2.7143, -38.1429)
  line L45 (2.7143, -38.1429) -> (5.7143, -38.1429)
  line L46 (5.7143, -38.1429) -> (5.7143, -41.1429)
  line L47 (5.7143, -41.1429) -> (2.7143, -41.1429)
  line L48 (-5.7143, -41.1429) -> (-5.7143, -38.1429)
  line L49 (-5.7143, -38.1429) -> (-2.7143, -38.1429)
  line L50 (-2.7143, -38.1429) -> (-2.7143, -41.1429)
  line L51 (-2.7143, -41.1429) -> (-5.7143, -41.1429)
  line L52 (-14.1429, -41.1429) -> (-14.1429, -38.1429)
  line L53 (-14.1429, -38.1429) -> (-11.1429, -38.1429)
  line L54 (-11.1429, -38.1429) -> (-11.1429, -41.1429)
  line L55 (-11.1429, -41.1429) -> (-14.1429, -41.1429)
  line L56 (-22.5714, -41.1429) -> (-22.5714, -38.1429)
  line L57 (-22.5714, -38.1429) -> (-19.5714, -38.1429)
  line L58 (-19.5714, -38.1429) -> (-19.5714, -41.1429)
  line L59 (-19.5714, -41.1429) -> (-22.5714, -41.1429)
  line L60 (-31, -41.1429) -> (-31, -38.1429)
  line L61 (-31, -38.1429) -> (-28, -38.1429)
  line L62 (-28, -38.1429) -> (-28, -41.1429)
  line L63 (-28, -41.1429) -> (-31, -41.1429)
  line L64 (28, -49.2857) -> (28, -46.2857)
  line L65 (28, -46.2857) -> (31, -46.2857)
  line L66 (31, -46.2857) -> (31, -49.2857)
  line L67 (31, -49.2857) -> (28, -49.2857)
  line L68 (19.5714, -49.2857) -> (19.5714, -46.2857)
  line L69 (19.5714, -46.2857) -> (22.5714, -46.2857)
  line L70 (22.5714, -46.2857) -> (22.5714, -49.2857)
  line L71 (22.5714, -49.2857) -> (19.5714, -49.2857)
  line L72 (11.1429, -49.2857) -> (11.1429, -46.2857)
  line L73 (11.1429, -46.2857) -> (14.1429, -46.2857)
  line L74 (14.1429, -46.2857) -> (14.1429, -49.2857)
  line L75 (14.1429, -49.2857) -> (11.1429, -49.2857)
  line L76 (2.7143, -49.2857) -> (2.7143, -46.2857)
  line L77 (2.7143, -46.2857) -> (5.7143, -46.2857)
  line L78 (5.7143, -46.2857) -> (5.7143, -49.2857)
  line L79 (5.7143, -49.2857) -> (2.7143, -49.2857)
  line L80 (-5.7143, -49.2857) -> (-5.7143, -46.2857)
  line L81 (-5.7143, -46.2857) -> (-2.7143, -46.2857)
  line L82 (-2.7143, -46.2857) -> (-2.7143, -49.2857)
  line L83 (-2.7143, -49.2857) -> (-5.7143, -49.2857)
  line L84 (-14.1429, -49.2857) -> (-14.1429, -46.2857)
  line L85 (-14.1429, -46.2857) -> (-11.1429, -46.2857)
  line L86 (-11.1429, -46.2857) -> (-11.1429, -49.2857)
  line L87 (-11.1429, -49.2857) -> (-14.1429, -49.2857)
  line L88 (-22.5714, -49.2857) -> (-22.5714, -46.2857)
  line L89 (-22.5714, -46.2857) -> (-19.5714, -46.2857)
  line L90 (-19.5714, -46.2857) -> (-19.5714, -49.2857)
  line L91 (-19.5714, -49.2857) -> (-22.5714, -49.2857)
  line L92 (-31, -49.2857) -> (-31, -46.2857)
  line L93 (-31, -46.2857) -> (-28, -46.2857)
  line L94 (-28, -46.2857) -> (-28, -49.2857)
  line L95 (-28, -49.2857) -> (-31, -49.2857)
  line L96 (28, -57.4286) -> (28, -54.4286)
  line L97 (28, -54.4286) -> (31, -54.4286)
  line L98 (31, -54.4286) -> (31, -57.4286)
  line L99 (31, -57.4286) -> (28, -57.4286)
  line L100 (19.5714, -57.4286) -> (19.5714, -54.4286)
  line L101 (19.5714, -54.4286) -> (22.5714, -54.4286)
  line L102 (22.5714, -54.4286) -> (22.5714, -57.4286)
  line L103 (22.5714, -57.4286) -> (19.5714, -57.4286)
  line L104 (11.1429, -57.4286) -> (11.1429, -54.4286)
  line L105 (11.1429, -54.4286) -> (14.1429, -54.4286)
  line L106 (14.1429, -54.4286) -> (14.1429, -57.4286)
  line L107 (14.1429, -57.4286) -> (11.1429, -57.4286)
  line L108 (2.7143, -57.4286) -> (2.7143, -54.4286)
  line L109 (2.7143, -54.4286) -> (5.7143, -54.4286)
  line L110 (5.7143, -54.4286) -> (5.7143, -57.4286)
  line L111 (5.7143, -57.4286) -> (2.7143, -57.4286)
  line L112 (-5.7143, -57.4286) -> (-5.7143, -54.4286)
  line L113 (-5.7143, -54.4286) -> (-2.7143, -54.4286)
  line L114 (-2.7143, -54.4286) -> (-2.7143, -57.4286)
  line L115 (-2.7143, -57.4286) -> (-5.7143, -57.4286)
  line L116 (-14.1429, -57.4286) -> (-14.1429, -54.4286)
  line L117 (-14.1429, -54.4286) -> (-11.1429, -54.4286)
  line L118 (-11.1429, -54.4286) -> (-11.1429, -57.4286)
  line L119 (-11.1429, -57.4286) -> (-14.1429, -57.4286)
  line L120 (-22.5714, -57.4286) -> (-22.5714, -54.4286)
  line L121 (-22.5714, -54.4286) -> (-19.5714, -54.4286)
  line L122 (-19.5714, -54.4286) -> (-19.5714, -57.4286)
  line L123 (-19.5714, -57.4286) -> (-22.5714, -57.4286)
  line L124 (-31, -57.4286) -> (-31, -54.4286)
  line L125 (-31, -54.4286) -> (-28, -54.4286)
  line L126 (-28, -54.4286) -> (-28, -57.4286)
  line L127 (-28, -57.4286) -> (-31, -57.4286)
  line L128 (28, -65.5714) -> (28, -62.5714)
  line L129 (28, -62.5714) -> (31, -62.5714)
  line L130 (31, -62.5714) -> (31, -65.5714)
  line L131 (31, -65.5714) -> (28, -65.5714)
  line L132 (19.5714, -65.5714) -> (19.5714, -62.5714)
  line L133 (19.5714, -62.5714) -> (22.5714, -62.5714)
  line L134 (22.5714, -62.5714) -> (22.5714, -65.5714)
  line L135 (22.5714, -65.5714) -> (19.5714, -65.5714)
  line L136 (11.1429, -65.5714) -> (11.1429, -62.5714)
  line L137 (11.1429, -62.5714) -> (14.1429, -62.5714)
  line L138 (14.1429, -62.5714) -> (14.1429, -65.5714)
  line L139 (14.1429, -65.5714) -> (11.1429, -65.5714)
  line L140 (2.7143, -65.5714) -> (2.7143, -62.5714)
  line L141 (2.7143, -62.5714) -> (5.7143, -62.5714)
  line L142 (5.7143, -62.5714) -> (5.7143, -65.5714)
  line L143 (5.7143, -65.5714) -> (2.7143, -65.5714)
  line L144 (-5.7143, -65.5714) -> (-5.7143, -62.5714)
  line L145 (-5.7143, -62.5714) -> (-2.7143, -62.5714)
  line L146 (-2.7143, -62.5714) -> (-2.7143, -65.5714)
  line L147 (-2.7143, -65.5714) -> (-5.7143, -65.5714)
  line L148 (-14.1429, -65.5714) -> (-14.1429, -62.5714)
  line L149 (-14.1429, -62.5714) -> (-11.1429, -62.5714)
  line L150 (-11.1429, -62.5714) -> (-11.1429, -65.5714)
  line L151 (-11.1429, -65.5714) -> (-14.1429, -65.5714)
  line L152 (-22.5714, -65.5714) -> (-22.5714, -62.5714)
  line L153 (-22.5714, -62.5714) -> (-19.5714, -62.5714)
  line L154 (-19.5714, -62.5714) -> (-19.5714, -65.5714)
  line L155 (-19.5714, -65.5714) -> (-22.5714, -65.5714)
  line L156 (-31, -65.5714) -> (-31, -62.5714)
  line L157 (-31, -62.5714) -> (-28, -62.5714)
  line L158 (-28, -62.5714) -> (-28, -65.5714)
  line L159 (-28, -65.5714) -> (-31, -65.5714)
  line L160 (28, -73.7143) -> (28, -70.7143)
  line L161 (28, -70.7143) -> (31, -70.7143)
  line L162 (31, -70.7143) -> (31, -73.7143)
  line L163 (31, -73.7143) -> (28, -73.7143)
  line L164 (19.5714, -73.7143) -> (19.5714, -70.7143)
  line L165 (19.5714, -70.7143) -> (22.5714, -70.7143)
  line L166 (22.5714, -70.7143) -> (22.5714, -73.7143)
  line L167 (22.5714, -73.7143) -> (19.5714, -73.7143)
  line L168 (11.1429, -73.7143) -> (11.1429, -70.7143)
  line L169 (11.1429, -70.7143) -> (14.1429, -70.7143)
  line L170 (14.1429, -70.7143) -> (14.1429, -73.7143)
  line L171 (14.1429, -73.7143) -> (11.1429, -73.7143)
  line L172 (2.7143, -73.7143) -> (2.7143, -70.7143)
  line L173 (2.7143, -70.7143) -> (5.7143, -70.7143)
  line L174 (5.7143, -70.7143) -> (5.7143, -73.7143)
  line L175 (5.7143, -73.7143) -> (2.7143, -73.7143)
  line L176 (-5.7143, -73.7143) -> (-5.7143, -70.7143)
  line L177 (-5.7143, -70.7143) -> (-2.7143, -70.7143)
  line L178 (-2.7143, -70.7143) -> (-2.7143, -73.7143)
  line L179 (-2.7143, -73.7143) -> (-5.7143, -73.7143)
  line L180 (-14.1429, -73.7143) -> (-14.1429, -70.7143)
  line L181 (-14.1429, -70.7143) -> (-11.1429, -70.7143)
  line L182 (-11.1429, -70.7143) -> (-11.1429, -73.7143)
  line L183 (-11.1429, -73.7143) -> (-14.1429, -73.7143)
  line L184 (-22.5714, -73.7143) -> (-22.5714, -70.7143)
  line L185 (-22.5714, -70.7143) -> (-19.5714, -70.7143)
  line L186 (-19.5714, -70.7143) -> (-19.5714, -73.7143)
  line L187 (-19.5714, -73.7143) -> (-22.5714, -73.7143)
  line L188 (-31, -73.7143) -> (-31, -70.7143)
  line L189 (-31, -70.7143) -> (-28, -70.7143)
  line L190 (-28, -70.7143) -> (-28, -73.7143)
  line L191 (-28, -73.7143) -> (-31, -73.7143)
  line L192 (28, -81.8571) -> (28, -78.8571)
  line L193 (28, -78.8571) -> (31, -78.8571)
  line L194 (31, -78.8571) -> (31, -81.8571)
  line L195 (31, -81.8571) -> (28, -81.8571)
  line L196 (19.5714, -81.8571) -> (19.5714, -78.8571)
  line L197 (19.5714, -78.8571) -> (22.5714, -78.8571)
  line L198 (22.5714, -78.8571) -> (22.5714, -81.8571)
  line L199 (22.5714, -81.8571) -> (19.5714, -81.8571)
  line L200 (11.1429, -81.8571) -> (11.1429, -78.8571)
  line L201 (11.1429, -78.8571) -> (14.1429, -78.8571)
  line L202 (14.1429, -78.8571) -> (14.1429, -81.8571)
  line L203 (14.1429, -81.8571) -> (11.1429, -81.8571)
  line L204 (2.7143, -81.8571) -> (2.7143, -78.8571)
  line L205 (2.7143, -78.8571) -> (5.7143, -78.8571)
  line L206 (5.7143, -78.8571) -> (5.7143, -81.8571)
  line L207 (5.7143, -81.8571) -> (2.7143, -81.8571)
  line L208 (-5.7143, -81.8571) -> (-5.7143, -78.8571)
  line L209 (-5.7143, -78.8571) -> (-2.7143, -78.8571)
  line L210 (-2.7143, -78.8571) -> (-2.7143, -81.8571)
  line L211 (-2.7143, -81.8571) -> (-5.7143, -81.8571)
  line L212 (-14.1429, -81.8571) -> (-14.1429, -78.8571)
  line L213 (-14.1429, -78.8571) -> (-11.1429, -78.8571)
  line L214 (-11.1429, -78.8571) -> (-11.1429, -81.8571)
  line L215 (-11.1429, -81.8571) -> (-14.1429, -81.8571)
  line L216 (-22.5714, -81.8571) -> (-22.5714, -78.8571)
  line L217 (-22.5714, -78.8571) -> (-19.5714, -78.8571)
  line L218 (-19.5714, -78.8571) -> (-19.5714, -81.8571)
  line L219 (-19.5714, -81.8571) -> (-22.5714, -81.8571)
  line L220 (-31, -81.8571) -> (-31, -78.8571)
  line L221 (-31, -78.8571) -> (-28, -78.8571)
  line L222 (-28, -78.8571) -> (-28, -81.8571)
  line L223 (-28, -81.8571) -> (-31, -81.8571)
  line L224 (28, -90) -> (28, -87)
  line L225 (28, -87) -> (31, -87)
  line L226 (31, -87) -> (31, -90)
  line L227 (31, -90) -> (28, -90)
  line L228 (19.5714, -90) -> (19.5714, -87)
  line L229 (19.5714, -87) -> (22.5714, -87)
  line L230 (22.5714, -87) -> (22.5714, -90)
  line L231 (22.5714, -90) -> (19.5714, -90)
  line L232 (11.1429, -90) -> (11.1429, -87)
  line L233 (11.1429, -87) -> (14.1429, -87)
  line L234 (14.1429, -87) -> (14.1429, -90)
  line L235 (14.1429, -90) -> (11.1429, -90)
  line L236 (2.7143, -90) -> (2.7143, -87)
  line L237 (2.7143, -87) -> (5.7143, -87)
  line L238 (5.7143, -87) -> (5.7143, -90)
  line L239 (5.7143, -90) -> (2.7143, -90)
  line L240 (-5.7143, -90) -> (-5.7143, -87)
  line L241 (-5.7143, -87) -> (-2.7143, -87)
  line L242 (-2.7143, -87) -> (-2.7143, -90)
  line L243 (-2.7143, -90) -> (-5.7143, -90)
  line L244 (-14.1429, -90) -> (-14.1429, -87)
  line L245 (-14.1429, -87) -> (-11.1429, -87)
  line L246 (-11.1429, -87) -> (-11.1429, -90)
  line L247 (-11.1429, -90) -> (-14.1429, -90)
  line L248 (-22.5714, -90) -> (-22.5714, -87)
  line L249 (-22.5714, -87) -> (-19.5714, -87)
  line L250 (-19.5714, -87) -> (-19.5714, -90)
  line L251 (-19.5714, -90) -> (-22.5714, -90)
  line L252 (-31, -90) -> (-31, -87)
  line L253 (-31, -87) -> (-28, -87)
  line L254 (-28, -87) -> (-28, -90)
  line L255 (-28, -90) -> (-31, -90)
  line L256 (-12, -19) -> (-26, -19)
  line L257 (-26, -19) -> (-26, -5)
  line L258 (-26, -5) -> (-12, -5)
  line L259 (-12, -5) -> (-12, -19)
  line L260 (26, -19) -> (12, -19)
  line L261 (12, -19) -> (12, -5)
  line L262 (12, -5) -> (26, -5)
  line L263 (26, -5) -> (26, -19)
  line L264 (7, -19) -> (-7, -19)
  line L265 (-7, -19) -> (-7, -5)
  line L266 (-7, -5) -> (7, -5)
  line L267 (7, -5) -> (7, -19)
  circle A0 centre (37.45, -25) radius 1.55
  circle A1 centre (37.45, -95) radius 1.55
  circle A2 centre (-37.45, -25) radius 1.55
  circle A3 centre (-37.45, -95) radius 1.55
  line L268 (-37.45, -100) -> (37.45, -100)
  arc A4 (37.45, -100) -> (42.45, -95) centre (37.45, -95) ccw
  line L269 (42.45, -95) -> (42.45, -5)
  arc A5 (42.45, -5) -> (37.45, 0) centre (37.45, -5) ccw
  line L270 (37.45, 0) -> (-37.45, 0)
  arc A6 (-37.45, 0) -> (-42.45, -5) centre (-37.45, -5) ccw
  line L271 (-42.45, -5) -> (-42.45, -95)
  arc A7 (-42.45, -95) -> (-37.45, -100) centre (-37.45, -95) ccw
extrude "Extrude1''''" add sketch "Sketch1 (4)" against normal blind 60 separate body contours L0 L1 L2 L3 | L4 L5 L6 L7 | L8 L9 L10 L11 | L12 L13 L14 L15 | L16 L17 L18 L19 | L20 L21 L22 L23 | L24 L25 L26 L27 | L28 L29 L30 L31 | L32 L33 L34 L35 | L36 L37 L38 L39 | L40 L41 L42 L43 | L44 L45 L46 L47 | L48 L49 L50 L51 | L52 L53 L54 L55 | L56 L57 L58 L59 | L60 L61 L62 L63 | L64 L65 L66 L67 | L68 L69 L70 L71 | L72 L73 L74 L75 | L76 L77 L78 L79 | L80 L81 L82 L83 | L84 L85 L86 L87 | L88 L89 L90 L91 | L92 L93 L94 L95 | L96 L97 L98 L99 | L100 L101 L102 L103 | L104 L105 L106 L107 | L108 L109 L110 L111 | L112 L113 L114 L115 | L116 L117 L118 L119 | L120 L121 L122 L123 | L124 L125 L126 L127 | L128 L129 L130 L131 | L132 L133 L134 L135 | L136 L137 L138 L139 | L140 L141 L142 L143 | L144 L145 L146 L147 | L148 L149 L150 L151 | L152 L153 L154 L155 | L156 L157 L158 L159 | L160 L161 L162 L163 | L164 L165 L166 L167 | L168 L169 L170 L171 | L172 L173 L174 L175 | L176 L177 L178 L179 | L180 L181 L182 L183 | L184 L185 L186 L187 | L188 L189 L190 L191 | L192 L193 L194 L195 | L196 L197 L198 L199 | L200 L201 L202 L203 | L204 L205 L206 L207 | L208 L209 L210 L211 | L212 L213 L214 L215 | L216 L217 L218 L219 | L220 L221 L222 L223 | L224 L225 L226 L227 | L228 L229 L230 L231 | L232 L233 L234 L235 | L236 L237 L238 L239 | L240 L241 L242 L243 | L244 L245 L246 L247 | L248 L249 L250 L251 | L252 L253 L254 L255 makes body 5 at (29, 87, 39) makes body 6 at (11.1429, 72.7143, 39) makes body 7 at (19.5714, 64.5714, 39) makes body 8 at (28, 56.4286, 39) makes body 9 at (11.1429, 40.1429, 39) makes body 10 at (19.5714, 32, 39) makes body 11 at (2.7143, 48.2857, 39) makes body 12 at (3.7143, 78.8571, 39) makes body 13 at (-5.7143, 72.7143, 39) makes body 14 at (-5.7143, 40.1429, 39) makes body 15 at (-14.1429, 48.2857, 39) makes body 16 at (-13.1429, 78.8571, 39) makes body 17 at (-22.5714, 72.7143, 39) makes body 18 at (-22.5714, 40.1429, 39) makes body 19 at (-31, 48.2857, 39) makes body 20 at (-30, 78.8571, 39) makes body 21 at (-31, 72.7143, 39) makes body 22 at (-31, 40.1429, 39) makes body 23 at (-22.5714, 48.2857, 39) makes body 24 at (-21.5714, 78.8571, 39) makes body 25 at (-14.1429, 72.7143, 39) makes body 26 at (-14.1429, 40.1429, 39) makes body 27 at (-5.7143, 48.2857, 39) makes body 28 at (-4.7143, 78.8571, 39) makes body 29 at (2.7143, 72.7143, 39) makes body 30 at (2.7143, 40.1429, 39) makes body 31 at (28, 32, 39) makes body 32 at (11.1429, 48.2857, 39) makes body 33 at (19.5714, 56.4286, 39) makes body 34 at (28, 64.5714, 39) makes body 35 at (12.1429, 78.8571, 39) makes body 36 at (20.5714, 87, 39) makes body 37 at (29, 78.8571, 39) makes body 38 at (19.5714, 72.7143, 39) makes body 39 at (11.1429, 64.5714, 39) makes body 40 at (28, 48.2857, 39) makes body 41 at (19.5714, 40.1429, 39) makes body 42 at (11.1429, 32, 39) makes body 43 at (2.7143, 56.4286, 39) makes body 44 at (3.7143, 87, 39) makes body 45 at (-5.7143, 64.5714, 39) makes body 46 at (-5.7143, 32, 39) makes body 47 at (-14.1429, 56.4286, 39) makes body 48 at (-13.1429, 87, 39) makes body 49 at (-22.5714, 64.5714, 39) makes body 50 at (-22.5714, 32, 39) makes body 51 at (-31, 56.4286, 39) makes body 52 at (-30, 87, 39) makes body 53 at (-31, 64.5714, 39) makes body 54 at (-31, 32, 39) makes body 55 at (-22.5714, 56.4286, 39) makes body 56 at (-21.5714, 87, 39) makes body 57 at (-14.1429, 64.5714, 39) makes body 58 at (-14.1429, 32, 39) makes body 59 at (-5.7143, 56.4286, 39) makes body 60 at (-4.7143, 87, 39) makes body 61 at (2.7143, 64.5714, 39) makes body 62 at (2.7143, 32, 39) makes body 63 at (28, 40.1429, 39) makes body 64 at (19.5714, 48.2857, 39) makes body 65 at (11.1429, 56.4286, 39) makes body 66 at (28, 72.7143, 39) makes body 67 at (20.5714, 78.8571, 39) makes body 68 at (12.1429, 87, 39) in component "Light Sticks"
component "Base" placed x (1, 0, 0) y (0, 1, 0) z (0, 0, 1) at (0, 0, 0)
component "Cover" placed x (1, 0, 0) y (0, 1, 0) z (0, 0, 1) at (0, 0, 0)
component "Layer" placed x (1, 0, 0) y (0, 1, 0) z (0, 0, 1) at (0, 0, 0)
component "Top" placed x (1, 0, 0) y (0, 1, 0) z (0, 0, 1) at (0, 0, 0)
component "Light Sticks" placed x (1, 0, 0) y (0, 1, 0) z (0, 0, 1) at (0, 0, 0)
equation "matrixLED_x = 63.7 mm" comment "1st LED to last LED in X-Direction"
equation "matrixLED_y = 61.7 mm" comment "1st LED to last LED in Y-Direction"
equation "matrix_length = 66.7 mm + 0.2 mm" comment "Matrix Board Length"
equation "matrix_width = 65.7 mm + 0.2 mm" comment "Matrix Board Width"
equation "length = 84.9 mm" comment "Base Length"
equation "width = 100 mm" comment "Base Width"
equation "height = 19 mm" comment "Base Height"
equation "thickness = 3 mm"
equation "wall = 5 mm" comment "Base Wall Thickness"
equation "nano_length = 17.6 mm"
equation "nano_width = 42.8 mm + 0.2 mm"
equation "nano_support = 4 mm"
equation "usb_length = 7.6 mm + 0.2 mm"
equation "usb_thickness = 3.9 mm + 0.2 mm"
equation "mic_length = 13.3 mm"
equation "mic_width = 20.5 mm"
equation "mic_diameter = 9.6 mm + 0.4 mm"
equation "d18 = length"
equation "d19 = width"
equation "d20 = height"
equation "d22 = matrix_length"
equation "d23 = wall"
equation "d24 = d23"
equation "d27 = -3.1 mm - 0.2 mm"
equation "d31 = mic_diameter"
equation "d32 = 2.5 mm + d31 / 2 + 0.2 mm"
equation "d39 = d35"
equation "d40 = usb_length"
equation "d41 = usb_thickness"
equation "d49 = nano_support"
equation "d51 = nano_width"
equation "d65 = 1.8 mm + d31 / 2 + 0.4 mm"
equation "d72 = thickness"
equation "switch_hole = 13.8 mm + 0.2 mm"
equation "switch_num = 3"
equation "switch_spacing = 19 mm"
equation "d77 = switch_hole"
equation "d78 = wall"
equation "d79 = matrixLED_x"
equation "d80 = matrixLED_y"
equation "d81 = thickness"
equation "d83 = d82"
equation "d86 = switch_num"
equation "d88 = switch_spacing"
equation "d91 = LED_num"
equation "d92 = LED_num"
equation "d93 = matrixLED_x - LED_size"
equation "d94 = matrixLED_y - LED_size"
equation "LED_size = 4.7 mm"
equation "LED_num = 8"
equation "d101 = thickness"
equation "d108 = thickness"
equation "d112 = ( 70 mm - matrix_width ) / 2"
